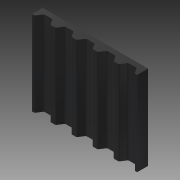
# Autodesk Inventor part: T2.5 belt-01
Saved by Autodesk Inventor 2015 SP1 (Build 190203100, 203)
## iProperties
Created: 2015-04-24
Part Number: T2.5 belt-01
Material: Rubber
Document SubType Name: Modeling
Designer: ubik
Density: 0.93 g/cm^3
Appearance: Rubber - Black - Version 1.1
Author: ubik
Autodesk Inventor part; units mm, degrees
ref_plane "YZ Plane" through (0, 0, 0) normal (1, 0, 0) x (0, 1, 0)
ref_plane "XZ Plane" through (0, 0, 0) normal (0, 1, 0) x (-1, 0, 0)
ref_plane "XY Plane" through (0, 0, 0) normal (0, 0, 1) x (1, 0, 0)
sketch "Sketch1" plane through (0, 0, 0) normal (0, 0, 1) x (1, 0, 0)
  line L0 (10, 0) -> (10.1908, 0)
  line L1 (10.359, 0.0918) -> (10.691, 0.6082)
  line L2 (11.809, 0.6082) -> (12.141, 0.0918)
  line L3 (10.8592, 0.7) -> (11.6408, 0.7)
  arc A0 (11.809, 0.6082) -> (11.6408, 0.7) centre (11.6408, 0.5) ccw
  arc A1 (10.8592, 0.7) -> (10.691, 0.6082) centre (10.8592, 0.5) ccw
  line L4 (12.3092, 0) -> (12.5, 0)
  arc A2 (10.1908, 0) -> (10.359, 0.0918) centre (10.1908, 0.2) ccw
  arc A3 (12.141, 0.0918) -> (12.3092, 0) centre (12.3092, 0.2) ccw
  line L5 (7.5, 0) -> (7.6908, 0)
  line L6 (7.859, 0.0918) -> (8.191, 0.6082)
  line L7 (9.309, 0.6082) -> (9.641, 0.0918)
  line L8 (8.3592, 0.7) -> (9.1408, 0.7)
  arc A4 (9.309, 0.6082) -> (9.1408, 0.7) centre (9.1408, 0.5) ccw
  arc A5 (8.3592, 0.7) -> (8.191, 0.6082) centre (8.3592, 0.5) ccw
  line L9 (9.8092, 0) -> (10, 0)
  arc A6 (7.6908, 0) -> (7.859, 0.0918) centre (7.6908, 0.2) ccw
  arc A7 (9.641, 0.0918) -> (9.8092, 0) centre (9.8092, 0.2) ccw
  line L10 (5, 0) -> (5.1908, 0)
  line L11 (5.359, 0.0918) -> (5.691, 0.6082)
  line L12 (6.809, 0.6082) -> (7.141, 0.0918)
  line L13 (5.8592, 0.7) -> (6.6408, 0.7)
  arc A8 (6.809, 0.6082) -> (6.6408, 0.7) centre (6.6408, 0.5) ccw
  arc A9 (5.8592, 0.7) -> (5.691, 0.6082) centre (5.8592, 0.5) ccw
  line L14 (7.3092, 0) -> (7.5, 0)
  arc A10 (5.1908, 0) -> (5.359, 0.0918) centre (5.1908, 0.2) ccw
  arc A11 (7.141, 0.0918) -> (7.3092, 0) centre (7.3092, 0.2) ccw
  line L15 (2.5, 0) -> (2.6908, 0)
  line L16 (2.859, 0.0918) -> (3.191, 0.6082)
  line L17 (4.309, 0.6082) -> (4.641, 0.0918)
  line L18 (3.3592, 0.7) -> (4.1408, 0.7)
  arc A12 (4.309, 0.6082) -> (4.1408, 0.7) centre (4.1408, 0.5) ccw
  arc A13 (3.3592, 0.7) -> (3.191, 0.6082) centre (3.3592, 0.5) ccw
  line L19 (4.8092, 0) -> (5, 0)
  arc A14 (2.6908, 0) -> (2.859, 0.0918) centre (2.6908, 0.2) ccw
  arc A15 (4.641, 0.0918) -> (4.8092, 0) centre (4.8092, 0.2) ccw
  line L20 (0, 0) -> (0.1908, 0)
  line L21 (0.359, 0.0918) -> (0.691, 0.6082)
  line L22 (1.809, 0.6082) -> (2.141, 0.0918)
  line L23 (0.8592, 0.7) -> (1.6408, 0.7)
  arc A16 (1.809, 0.6082) -> (1.6408, 0.7) centre (1.6408, 0.5) ccw
  arc A17 (0.8592, 0.7) -> (0.691, 0.6082) centre (0.8592, 0.5) ccw
  line L24 (2.3092, 0) -> (2.5, 0)
  arc A18 (0.1908, 0) -> (0.359, 0.0918) centre (0.1908, 0.2) ccw
  arc A19 (2.141, 0.0918) -> (2.3092, 0) centre (2.3092, 0.2) ccw
  line L25 (12.5, 0) -> (12.5, 1.3)
  line L26 (12.5, 1.3) -> (0, 1.3)
  line L27 (0, 1.3) -> (0, 0)
  line L28 (7.3092, 0) -> (7.6908, 0)
  line L29 (9.8092, 0) -> (10.1908, 0)
  line L30 (12.3092, 0) -> (12.5, 0)
  line L31 (4.8092, 0) -> (5.1908, 0)
  line L32 (0, 0) -> (0.1908, 0)
  line L33 (2.3092, 0) -> (2.6908, 0)
  point P0 (0, 0)
  point P1 (10.3, 0)
  point P2 (12.2, 0)
  point P3 (7.8, 0)
  point P4 (9.7, 0)
  point P5 (5.3, 0)
  point P6 (7.2, 0)
  point P7 (2.8, 0)
  point P8 (4.7, 0)
  point P9 (0.3, 0)
  point P10 (2.2, 0)
  dimension "d14" = 10
  dimension "d5" = 0.3
  dimension "d7" = 0.2
  dimension "d8" = 0.2
  dimension "d11" = 2.5
  dimension "d16" = 1.3
  constraints: 68 end point, 40 point on circle, 20 centre point, 20 point on line, 8 tangent, 7 parallel, 6 horizontal, 6 perpendicular, 2 equal radius
  measures "d5" distance of L0.start point (10.3, 0)
  measures "d7" radius of A0
  measures "d8" radius of A2
  measures "d11" distance of L0.start L5.start
  measures "d16" distance of L25.end L25.start
extrude "Extrusion1" add sketch "Sketch1" along normal blind 10
pattern_of_one "Rectangular Pattern1"
body "Solid1"
